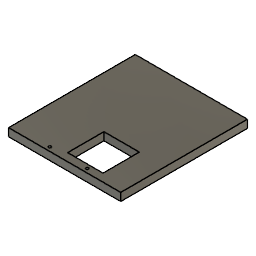
rightside (Autodesk Fusion 360 design; units mm, degrees)
Autodesk Fusion 360 part; units mm, degrees
sketch "Skizze1" plane through (0, 0, 0) normal (0, 0, 1) x (1, 0, 0)
  line L0 (0, 0) -> (127, 0)
  line L1 (127, 0) -> (127, 143.5)
  line L2 (127, 143.5) -> (0, 143.5)
  line L3 (0, 143.5) -> (0, 0)
  line L4 (98, 50) -> (58, 50)
  line L5 (58, 50) -> (58, 9)
  line L6 (58, 9) -> (98, 9)
  line L7 (98, 9) -> (98, 50)
  circle A0 centre (84.6667, 4.5) radius 1.5
  circle A1 centre (42.3337, 4.5) radius 1.5
  dimension "d1" = 127
  dimension "d2" = 143.5
  dimension "d3" = 40
  dimension "d4" = 29
  dimension "d5" = 50
  dimension "d6" = 41
  dimension "d7" = 3
  dimension "d8" = 4.5
  dimension "d9" = 42.3333
  dimension "d10" = 3
  constraint horizontal L0
  constraint vertical L1
  constraint horizontal L2
  constraint vertical L3
  constraint coincident L0.start L3.end
  constraint perpendicular L3 L4
  constraint perpendicular L4 L5
  constraint perpendicular L5 L6
  constraint perpendicular L4 L7
  measures "d1" distance of L0.start L0.end
  measures "d2" distance of L0.start L2.end
  measures "d3" distance of L4.start L4.end
  measures "d4" distance of L1 L4.start
  measures "d5" distance of L0 L4
  measures "d6" distance of L4.end L5.end
  measures "d7" diameter of A0
  measures "d8" distance of L0 A0.centre
  measures "d9" distance of L1 A0.centre
  measures "d10" diameter of A1
extrude "Extrusion1" add sketch "Skizze1" along normal blind 9
equation "d5 = 41 mm + 9 mm"
equation "d8 = ( 9 / 2 ) * 1 mm"
equation "d9 = ( 127 / 3 ) * 1 mm"
